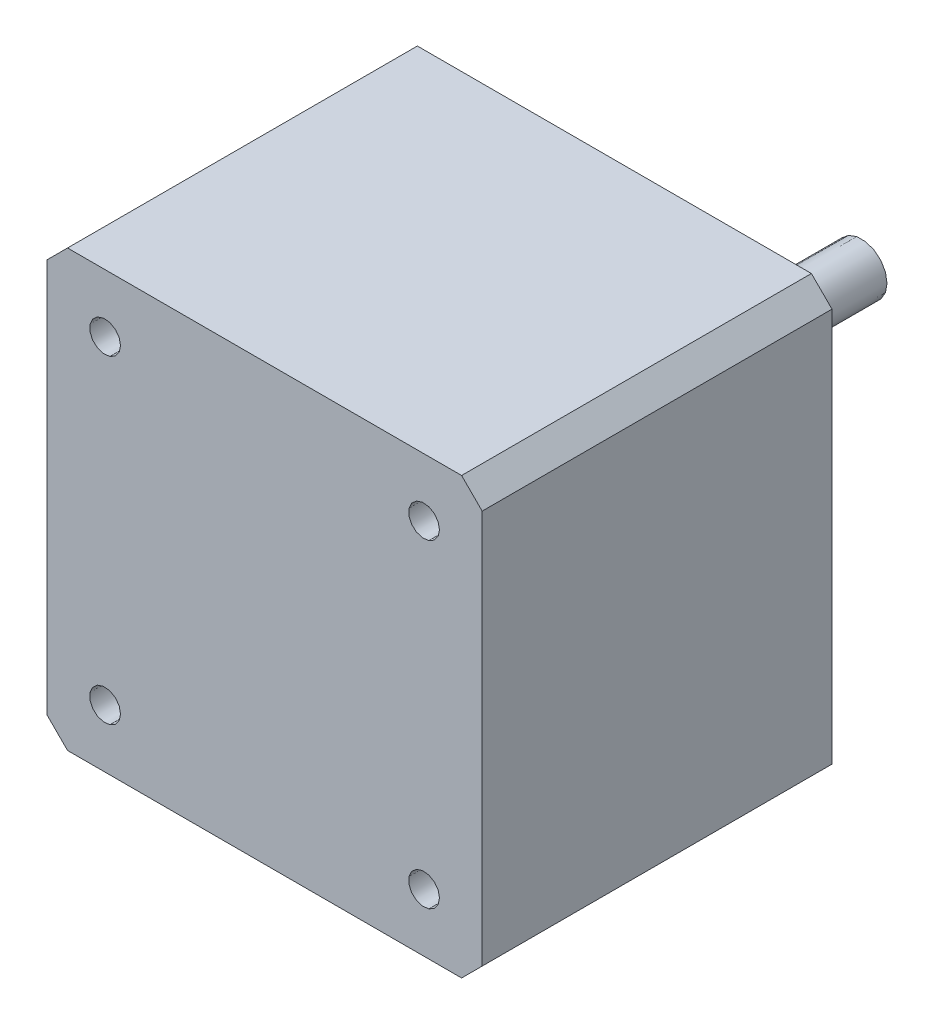
# Autodesk Inventor part: motor
Saved by Autodesk Inventor 2023 (Build 270158000, 158)
## iProperties
Created: 2022-07-02
Part Number: motor
Material: Generic
Document SubType Name: Modeling
Designer: Zayed
Density: 1 g/cm^3
Appearance: Default
Author: Zayed
Autodesk Inventor part; units mm, degrees
ref_plane "YZ Plane" through (0, 0, 0) normal (1, 0, 0) x (0, 1, 0)
ref_plane "XZ Plane" through (0, 0, 0) normal (0, 1, 0) x (-1, 0, 0)
ref_plane "XY Plane" through (0, 0, 0) normal (0, 0, 1) x (1, 0, 0)
sketch "body" plane through (0, 0, 0) normal (0, 0, 1) x (1, 0, 0)
  line L0 (-19.15, -21.15) -> (19.15, -21.15)
  line L1 (21.15, -19.15) -> (21.15, 19.15)
  line L2 (19.15, 21.15) -> (-19.15, 21.15)
  line L3 (-21.15, 19.15) -> (-21.15, -19.15)
  line L4 (-21.15, -21.15) -> (21.15, 21.15) construction
  line L5 (21.15, -21.15) -> (-21.15, 21.15) construction
  line L6 (-19.15, -21.15) -> (-21.15, -19.15)
  line L7 (-21.15, 19.15) -> (-19.15, 21.15)
  line L8 (21.15, 19.15) -> (19.15, 21.15)
  line L9 (19.15, -21.15) -> (21.15, -19.15)
  circle A0 centre (-15.5, 15.5) radius 1.5
  circle A1 centre (15.5, 15.5) radius 1.5
  circle A2 centre (15.5, -15.5) radius 1.5
  circle A3 centre (-15.5, -15.5) radius 1.5
  point P0 (0, 0)
  dimension "d5" = 42.3
  dimension "d6" = 42.3
  dimension "d7" = 2
  dimension "d8" = 2
  dimension "d9" = 2
  dimension "d10" = 2
  dimension "d11" = 2
  dimension "d12" = 2
  dimension "d13" = 2
  dimension "d14" = 2
  dimension "d15" = 3
  dimension "d16" = 3
  dimension "d17" = 3
  dimension "d18" = 3
  constraints: 20 end point, 11 point on line, 4 centre point, 2 midpoint, 2 parallel, 1 horizontal, 1 perpendicular
  measures "d5" distance of L5.end L4.end
  measures "d6" distance of L4.end L5.start
  measures "d7" distance of L0.start L4.start
  measures "d8" distance of L3.end L4.start
  measures "d9" distance of L3.start L5.end
  measures "d10" distance of L2.end L5.end
  measures "d11" distance of L1.end L4.end
  measures "d12" distance of L2.start L4.end
  measures "d13" distance of L0.end L5.start
  measures "d14" distance of L1.start L5.start
  measures "d15" diameter of A0
  measures "d16" diameter of A1
  measures "d17" diameter of A2
  measures "d18" diameter of A3
sketch "Sketch6" plane through (0, 0, 0) normal (0, 0, 1) x (1, 0, 0)
  circle A0 centre (0, 0) radius 2.5
  dimension "d19" = 5
  constraints: 1 centre point, 1 coincident
  measures "d19" diameter of A0
extrude "Extrusion1" add sketch "body" along normal blind 34
extrude "Extrusion2" add sketch "Sketch6" against normal blind 24
equation "\"d8\" = d7"
equation "\"d10\" = d9"
equation "\"d11\" = d9"
equation "\"d12\" = d11"
equation "\"d13\" = d9"
equation "\"d14\" = d13"
body "Solid1"
